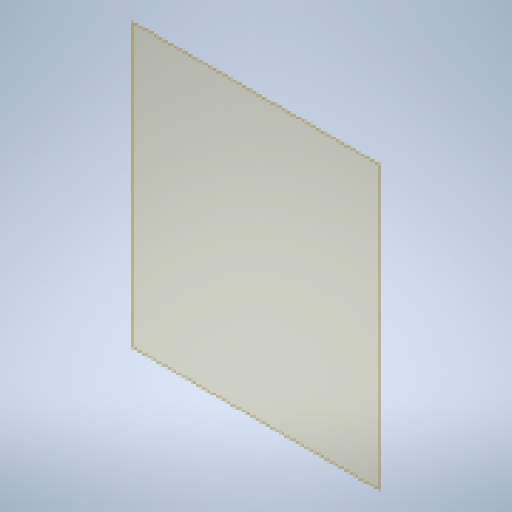
# Autodesk Inventor part: Part7
Saved by Autodesk Inventor 2025.2 (Build 292293000, 293)
## iProperties
Created: 2025-03-25
Part Number: Part7
Material: Steel, Mild
Document SubType Name: Modeling
Designer: bless
Density: 7.85 g/cm^3
Appearance: Semi-Polished
Author: bless
Autodesk Inventor part; units mm, degrees
ref_plane "YZ Plane" through (0, 0, 0) normal (1, 0, 0) x (0, 1, 0)
ref_plane "XZ Plane" through (0, 0, 0) normal (0, 1, 0) x (-1, 0, 0)
ref_plane "XY Plane" through (0, 0, 0) normal (0, 0, 1) x (1, 0, 0)
ref_plane "Work Plane1" through (0, 0, 0) normal (0, 0, 1) x (1, 0, 0)
sketch "Sketch1" plane through (0, 0, 0) normal (0, 0, 1) x (1, 0, 0)
  circle A0 centre (-23.3137, -216.6379) radius 30
  line L0 (-120.3137, -36.6379) -> (73.6863, -36.6379) projected
  line L1 (65.6863, -36.6379) -> (-112.3137, -36.6379) projected
  line L2 (-34.5156, -26.6379) -> (-173.1117, -26.6379) projected
  point P0 (0, 0)
  point P1 (-23.3137, -36.6379)
  dimension "d0" = 60
  dimension "d1" = 190
  constraints: 1 centre point, 1 midpoint, 1 vertical alignment
  measures "d0" diameter of A0
  measures "d1" distance from line of A0.centre L2
extrude "Extrusion1" add sketch "Sketch1" against normal blind 84.25
ref_plane "Work Plane2" through (-23.3137, -256.6379, -119.9996) normal (0, -1, 0) x (1, 0, 0)
sketch "Sketch2" plane through (-23.3137, -256.6379, -119.9996) normal (0, -1, 0) x (1, 0, 0)
  circle A0 centre (0, 0) radius 97 projected
  line L0 (-30, 35.7496) -> (30, 35.7496) projected
  line L1 (30, 119.9996) -> (-30, 119.9996) projected
  line L2 (-30, 119.9996) -> (-30, 35.7496) projected
  line L3 (30, 119.9996) -> (30, 35.7496) projected
  point P0 (23.3137, 119.9996)
  point P1 (30, 92.2442)
  point P2 (-30, 92.2442)
extrude "Extrusion2" cut sketch "Sketch2" against normal through all contours L3 L0 L2 A0 picked at (2.032, 56.1025)
body "Solid1"
